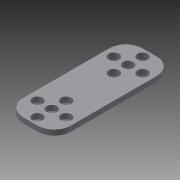
# Autodesk Inventor part: ArmToArm
Saved by Autodesk Inventor 2014 (Build 180170000, 170)
## iProperties
Created: 2014-03-07
Part Number: ArmToArm
Material: Générique
Document SubType Name: Modeling
Designer: Grégoire
Density: 1 g/cm^3
Appearance: Par défaut
Author: Grégoire
Autodesk Inventor part; units mm, degrees
ref_plane "YZ Plane" through (0, 0, 0) normal (1, 0, 0) x (0, 1, 0)
ref_plane "XZ Plane" through (0, 0, 0) normal (0, 1, 0) x (-1, 0, 0)
ref_plane "XY Plane" through (0, 0, 0) normal (0, 0, 1) x (1, 0, 0)
sketch "Esquisse5" plane through (0, 0, 0) normal (0, 0, 1) x (1, 0, 0)
  line L0 (0, 0) -> (20, 0)
  line L1 (20, 0) -> (20, 25)
  line L2 (20, 25) -> (0, 25)
  line L3 (0, 25) -> (0, 0)
  line L4 (10, 0) -> (10, 25) construction
  circle A0 centre (10, 3) radius 2.15
  circle A1 centre (10, 9) radius 2.15
  circle A2 centre (10, 15) radius 2.15
  line L5 (10, 9) -> (20, 9) construction
  circle A3 centre (16, 9) radius 2.15
  circle A4 centre (4, 9) radius 2.15
  circle A5 centre (10, 9) radius 2.15
  dimension "d61" = 20
  dimension "d62" = 25
  dimension "d63" = 3
  dimension "d64" = 4.3
  dimension "d67" = 6
  dimension "d74" = 6
  dimension "d77" = 6
  constraints: 12 end point, 6 centre point, 3 horizontal, 2 midpoint, 2 parallel, 2 perpendicular, 2 point on line, 1 vertical, 10 other
  measures "d61" distance of L0.start L0.end
  measures "d62" distance of L2.end L0.start
  measures "d63" distance from line of L0 A0.centre
  measures "d64" diameter of A0
  measures "d67" distance of A0.centre L5.start
  measures "d74" distance of L5.start A3.centre
  measures "d77" distance of L5.start A4.centre
extrude "Extrusion5" add sketch "Esquisse5" along normal blind 2.2
fillet "Congé4" radius 7 2 edges at (0, 0, 1.1) (20, 0, 1.1)
mirror "Symétrie1" about plane through (20, 25, 0) normal (0, 1, 0)
equation "\"d64\" = Holes"
equation "\"d80\" = Depth"
equation "\"d100\" = Rounding"
equation "\"Depth\" = 2.2"
equation "\"Holes\" = 4.3"
equation "\"Height\" = 0"
equation "\"Rounding\" = 7"
